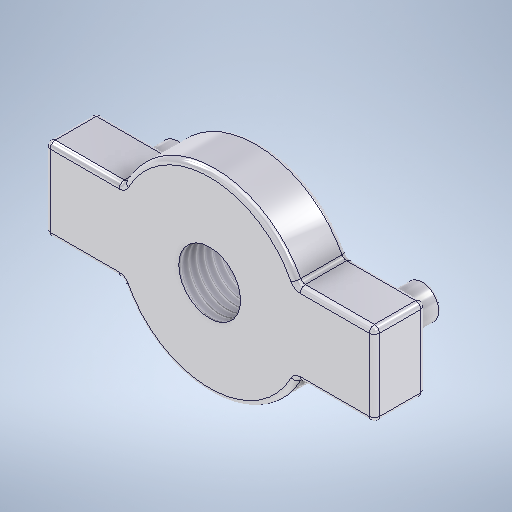
# Autodesk Inventor part: Steering Front
Saved by Autodesk Inventor 2025.2 (Build 292293000, 293)
## iProperties
Created: 2025-02-03
Part Number: Steering Front
Material: Generic
Document SubType Name: Modeling
Designer: eason
Density: 1 g/cm^3
Appearance: Opal
Author: eason
Autodesk Inventor part; units mm, degrees
ref_plane "YZ Plane" through (0, 0, 0) normal (1, 0, 0) x (0, 1, 0)
ref_plane "XZ Plane" through (0, 0, 0) normal (0, 1, 0) x (-1, 0, 0)
ref_plane "XY Plane" through (0, 0, 0) normal (0, 0, 1) x (1, 0, 0)
sketch "Sketch1" plane through (0, 0, 0) normal (0, 0, 1) x (1, 0, 0)
  circle A0 centre (0, 0) radius 6
  circle A1 centre (-23.75, 0) radius 3.25
  line L0 (-20.5, 0) -> (-20.5, 3.4324)
  line L1 (-27, 0) -> (-27, 3.2184)
  line L2 (-44.8, 0) -> (44.8, 0) projected
  line L3 (0, 26.25) -> (0, -26.25) projected
  circle A2 centre (23.75, 0) radius 3.25
  line L4 (32, 8) -> (32, -8)
  line L5 (-32, -8) -> (-32, 8)
  arc A3 (-16.9577, -8) -> (16.9577, -8) centre (0, 0) ccw
  arc A4 (16.9577, 8) -> (-16.9577, 8) centre (0, 0) ccw
  line L6 (32, -8) -> (16.9577, -8)
  line L7 (-16.9577, -8) -> (-32, -8)
  line L8 (-32, 8) -> (-16.9577, 8)
  line L9 (16.9577, 8) -> (32, 8)
  dimension "d0" = 12
  dimension "d4" = 20.5
  dimension "d5" = 27
  dimension "d9" = 5
  dimension "d10" = 18.75
  dimension "d11" = 18.75
  constraints: 16 end point, 6 point on circle, 5 centre point, 5 parallel, 3 perpendicular, 2 coincident, 2 horizontal, 2 tangent, 2 vertical, 1 point on line, 1 symmetric about line, 1 other
  measures "d0" diameter of A0
  measures "d4" distance between parallel lines of L3 L0
  measures "d5" distance between parallel lines of L3 L1
  measures "d9" distance between parallel lines of L5 L1
  measures "d10" radius of A4
  measures "d11" radius of A3
extrude "Extrusion1" add sketch "Sketch1" along normal blind 10 contours L2 A2 L4 L6 A3 L3 A0 | A0 L3 A4 L9 L4 L2 A2 | A0 L2 A1 L5 L8 A4 L3 | L3 A3 L7 L5 L2 A1 A0 | A2 L2 | L2 A2 | L2 A1 | A1 L2
extrude "Extrusion2" add sketch "Sketch1" against normal blind 8 contours A2 L2 | L2 A2 | L2 A1 | A1 L2
fillet "Fillet1" radius 1 24 edges at (0, 18.75, 10) (24.4788, 8, 10) (32, 0, 10) (24.4788, -8, 10) (0, -18.75, 10) (-24.4788, -8, 10) (-32, 0, 10) (-24.4788, 8, 10) (32, 0, 0) (24.4788, 8, 0) (0, 18.75, 0) (24.4788, -8, 0) (0, -18.75, 0) (-24.4788, -8, 0) (-24.4788, 8, 0) (-32, 0, 0) (-32, -8, 5) (-32, 8, 5) (32, 8, 5) (32, -8, 5) (16.9577, -8, 5) (-16.9577, -8, 5) (-16.9577, 8, 5) (16.9577, 8, 5)
fillet "Fillet3" radius 0.5 2 edges at (20.5, 0, -8) (-27, 0, -8)
thread "Thread1" size "M12x1.5" class "6H" standard "ANSI Metric M Profile" full length
body "Solid1"
